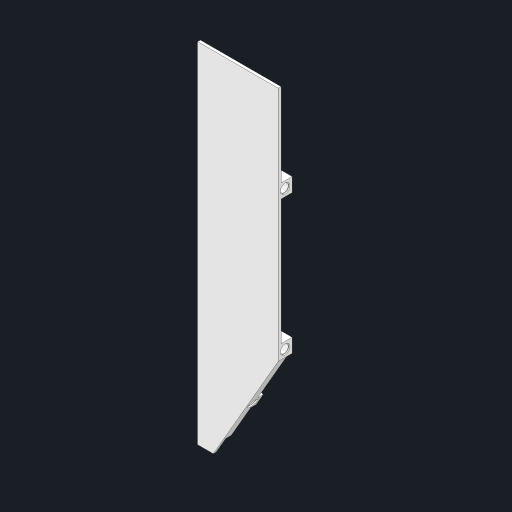
# Autodesk Inventor part: blank_side_r
Saved by Autodesk Inventor 2023 (Build 270158000, 158)
## iProperties
Created: 2024-05-25
Part Number: blank_side_r
Material: ABS Plastic
Document SubType Name: Modeling
Designer: szymo
Density: 1.06 g/cm^3
Appearance: Smooth - White
Mass: 11.6774 g
Surface Area: 101.879 cm^2
Volume: 11.0164 cm^3
Author: szymo
Autodesk Inventor part; units mm, degrees
ref_plane "YZ Plane" through (0, 0, 0) normal (1, 0, 0) x (0, 1, 0)
ref_plane "XZ Plane" through (0, 0, 0) normal (0, 1, 0) x (-1, 0, 0)
ref_plane "XY Plane" through (0, 0, 0) normal (0, 0, 1) x (1, 0, 0)
sketch "Sketch1" plane through (0, 0, 0) normal (0, 0, 1) x (1, 0, 0)
  line L0 (3.5, 3.5) -> (-1, 3.5) projected
  line L1 (-1, 3.5) -> (-1, -0.5) projected
  line L2 (-1, -0.5) -> (-4.5, -0.5) projected
  line L3 (-4.5, -0.5) -> (-4.5, -14.5) projected
  line L4 (-4.5, -14.5) -> (4.5, -0.5) projected
  line L5 (4.5, -0.5) -> (3.5, -0.5) projected
  line L6 (3.5, -0.5) -> (3.5, 3.5) projected
  circle A0 centre (13, 116) radius 15 projected
  line L7 (3.5, 3.5) -> (28, 45.9352)
  line L8 (28, 45.9352) -> (28, 131)
  line L9 (28, 131) -> (-1, 131)
  line L10 (-1, 131) -> (-1, 3.5)
  line L11 (-1, 5.5) -> (4.6547, 5.5)
  point P0 (0, 0)
  dimension "d1" = 30
  dimension "d7" = 2
  constraints: 10 end point, 2 horizontal, 2 point on line, 2 tangent, 2 vertical
  measures "d1" angle of L6 L7
  measures "d7" distance between parallel lines of L11 L0
extrude "Extrusion1" add sketch "Sketch1" against normal blind 1 contours L11 L10 A0 L8 L7 | L10 A0 | A0 L9 L8 | L10 L9 A0 picked at (14.8903, 120.4447)
sketch "Sketch3" plane through (0, 0, -1) normal (0, 0, -1) x (-1, 0, 0)
  line L0 (1, 13.25) -> (1, 15.75) projected
  line L1 (1, 15.75) -> (-2.9023, 15.75)
  line L2 (-2.9023, 15.75) -> (-2.9023, 13.25)
  line L3 (-2.9023, 13.25) -> (1, 13.25)
  line L4 (1, 13.25) -> (1, 15.75)
  line L5 (1, 5.5) -> (1, 131) projected
  line L6 (1, 11.5) -> (-4, 11.5)
  line L7 (-4, 11.5) -> (-4, 17.5)
  line L8 (-4, 17.5) -> (1, 17.5)
  line L9 (1, 17.5) -> (1, 11.5)
  line L10 (-4.6547, 5.5) -> (1, 5.5) projected
  line L11 (1, 5.5) -> (1, 131) projected
  line L12 (1, 131) -> (-28, 131) projected
  line L13 (-28, 131) -> (-28, 45.9352) projected
  line L14 (-28, 45.9352) -> (-4.6547, 5.5) projected
  line L15 (1, 20.5) -> (1, 3.5) projected
  line L16 (-4, 17.5) -> (1, 17.5)
  line L17 (1, 17.5) -> (1, 26.5)
  line L18 (1, 26.5) -> (-4, 26.5)
  line L19 (-4, 26.5) -> (-4, 17.5)
  point P0 (0, 0)
  point P1 (-2.9023, 14.5)
  point P2 (1, 17.5)
  dimension "d8" = 3
  dimension "d9" = 3
  dimension "d10" = 5
  dimension "d11" = 6
  constraints: 24 end point, 6 parallel, 3 horizontal, 3 perpendicular, 3 point on line, 1 midpoint, 1 other
  measures "d8" distance from line of L6 point (-2.902, 14.5)
  measures "d9" distance from line of L8 point (-2.902, 14.5)
  measures "d10" distance between parallel lines of L5 L7
  measures "d11" distance from line of L18 point (1, 20.5)
extrude "Extrusion2" add sketch "Sketch3" along normal blind 12 contours L3 L2 L1 L0 | L5 L6 L7 L8 L1 L2 L3
sketch "Sketch4" plane through (0, 0, -1) normal (0, 0, -1) x (-1, 0, 0)
  line L0 (-4, 11.5) -> (-4, 17.5) projected
  line L1 (1, 17.5) -> (1, 131) projected
  line L2 (1, 131) -> (-28, 131) projected
  line L3 (-28, 131) -> (-28, 45.9352) projected
  line L4 (-28, 45.9352) -> (-4.6547, 5.5) projected
  line L5 (-4.6547, 5.5) -> (1, 5.5) projected
  line L6 (1, 5.5) -> (1, 11.5) projected
  line L7 (-28, 45.9352) -> (-28, 50.9352)
  line L8 (-28, 50.9352) -> (-23, 50.9352)
  line L9 (-23, 50.9352) -> (-23, 45.9352)
  line L10 (-23, 45.9352) -> (-28, 45.9352)
  circle A0 centre (-13, 116) radius 15 projected
  line L11 (1, 131) -> (1, 5.5) projected
  line L12 (1, 101) -> (-28, 101)
  line L13 (-28, 101) -> (-23, 101)
  line L14 (-23, 101) -> (-23, 96)
  line L15 (-23, 96) -> (-28, 96)
  line L16 (-28, 96) -> (-28, 101)
  line L17 (-17.5774, 27.8827) -> (-15.0774, 23.5526)
  line L18 (-15.0774, 23.5526) -> (-10.7472, 26.0526)
  line L19 (-10.7472, 26.0526) -> (-13.2472, 30.3827)
  line L20 (-13.2472, 30.3827) -> (-17.5774, 27.8827)
  line L21 (1, 11.5) -> (-4, 11.5) projected
  line L22 (-4, 17.5) -> (1, 17.5) projected
  line L23 (1, 101) -> (-4, 101)
  line L24 (-4, 101) -> (-4, 96)
  line L25 (-4, 96) -> (1, 96)
  line L26 (1, 96) -> (1, 101)
  line L27 (1, 17.5) -> (-4, 17.5) projected
  line L28 (-4, 17.5) -> (-4, 11.5) projected
  line L29 (-4, 11.5) -> (1, 11.5) projected
  line L30 (1, 11.5) -> (1, 17.5) projected
  line L31 (1, 17.5) -> (-4, 17.5)
  line L32 (-4, 17.5) -> (-4, 22.5)
  line L33 (-4, 22.5) -> (1, 22.5)
  line L34 (1, 22.5) -> (1, 17.5)
  point P0 (0, 0)
  point P1 (1, 36.3564)
  point P2 (1, 96)
  dimension "d16" = 5
  dimension "d17" = 5
  dimension "d18" = 5
  dimension "d19" = 5
  dimension "d20" = 5
  dimension "d21" = 5
  dimension "d22" = 18.0526
  dimension "d23" = 18.0526
  dimension "d168" = 5
  dimension "d169" = 5
  dimension "d170" = 5
  dimension "d171" = 5
  constraints: 42 end point, 10 parallel, 5 perpendicular, 5 point on line, 4 horizontal, 1 tangent
  measures "d16" distance of L3.end L7.end
  measures "d17" distance of L7.end L8.end
  measures "d18" distance of L14.end L15.end
  measures "d19" distance of L13.end L14.end
  measures "d20" distance of L17.start L17.end
  measures "d21" distance of L18.end L17.end
  measures "d22" vertical distance of L17.end L4.end
  measures "d23" vertical distance of L3.end L17.start
  measures "d168" distance of L25.end L24.end
  measures "d169" distance of L24.end L23.end
  measures "d170" distance of L32.end L33.end
  measures "d171" distance of L31.end L32.end
extrude "forInserts" add sketch "Sketch4" along normal blind 4 contours L32 L33 L1 L22 | L25 L24 L12 L1 | L4 L20 L19 L18 | L3 L8 L9 L10 | L14 L15 L3 L12
sketch "Sketch5" plane through (0, 0, -1) normal (0, 0, -1) x (-1, 0, 0)
  line L0 (-28, 96) -> (-28, 50.9352) projected
  line L1 (-28, 50.9352) -> (-23, 50.9352) projected
  line L2 (-23, 50.9352) -> (-23, 45.9352) projected
  line L3 (-23, 45.9352) -> (-28, 45.9352) projected
  line L4 (-28, 45.9352) -> (-17.5774, 27.8827) projected
  line L5 (-17.5774, 27.8827) -> (-13.2472, 30.3827) projected
  line L6 (-13.2472, 30.3827) -> (-10.7472, 26.0526) projected
  line L7 (-10.7472, 26.0526) -> (-15.0774, 23.5526) projected
  line L8 (-15.0774, 23.5526) -> (-4.6547, 5.5) projected
  line L9 (-4.6547, 5.5) -> (1, 5.5) projected
  line L10 (1, 5.5) -> (1, 11.5) projected
  line L11 (-4, 11.5) -> (-4, 22.5) projected
  line L12 (1, 101) -> (1, 131) projected
  line L13 (1, 131) -> (-28, 131) projected
  line L14 (-28, 45.9352) -> (1, 45.9352)
  line L15 (1, 131) -> (1, 5.5) projected
  line L16 (-23, 50.9352) -> (1, 50.9352)
  arc A0 (-28, 101) -> (-26.5929, 101.3416) centre (-28, 104.0688) ccw
  line L17 (-28, 96) -> (1, 96)
  line L18 (-28, 101) -> (1, 101)
  line L19 (-23, 50.9352) -> (-23, 96)
  line L20 (-2, 96) -> (-2, 17.5)
  line L21 (-4, 11.5) -> (-8.1188, 11.5)
  line L22 (-2.3453, 11.5) -> (-22.2265, 45.9352)
  line L23 (-13.2472, 30.3827) -> (-2, 45.9352) construction
  line L24 (-11.8776, 28.0104) -> (-2, 41.669)
  line L25 (-5.0852, 45.9352) -> (-14.6169, 32.755)
  line L26 (1, 11.5) -> (-4, 11.5) projected
  line L27 (-28, 101) -> (-23, 101) projected
  line L28 (-23, 101) -> (-23, 96) projected
  line L29 (-23, 96) -> (-28, 96) projected
  line L30 (-4, 22.5) -> (1, 22.5) projected
  line L31 (1, 22.5) -> (1, 96) projected
  line L32 (1, 96) -> (-4, 96) projected
  line L33 (-4, 96) -> (-4, 101) projected
  line L34 (-4, 101) -> (1, 101) projected
  line L35 (-28, 131) -> (-28, 101) projected
  point P0 (0, 0)
  point P1 (1, 36.3564)
  point P2 (-2, 50.9352)
  point P3 (1, 101)
  point P4 (-4, 14.366)
  point P5 (1, 96)
  point P6 (1, 45.9352)
  point P7 (1, 101)
  point P8 (1, 45.9352)
  point P9 (-2, 22.5)
  point P10 (1, 50.9352)
  point P11 (1, 50.9352)
  dimension "d26" = 5
  dimension "d27" = 3
  dimension "d28" = 5
  dimension "d29" = 2.5
  dimension "d30" = 2.5
  constraints: 22 end point, 15 point on line, 4 parallel, 4 perpendicular, 2 point on circle, 1 centre point, 1 horizontal, 1 vertical
  measures "d26" distance between parallel lines of L14 L16
  measures "d27" distance between parallel lines of L20 L15
  measures "d28" distance between parallel lines of L4 L22
  measures "d29" distance between parallel lines of L23 L25
  measures "d30" distance between parallel lines of L23 L24
extrude "zeberka" add sketch "Sketch5" along normal blind 2 contours L28 L18 L33 L17 | L16 L20 L14 L2 | L14 L22 L5 L4 L3 | L20 L17 L15 L16 | L16 L15 L14 L20 | L20 L24 L6 L22 L25 L14 | L14 L15 L30 L20 | L15 L26 L22 L11 L30 | L22 L11 L21 L8 L7
sketch "Sketch9" plane through (-1, 5.5, 0) normal (-1, 0, 0) x (0, 0, 1)
  circle A0 centre (-9.5, 9) radius 1.25 projected
  point P0 (0, -5.5)
  constraints: 1 coincident
hole "Hole3" at (-1, 14.5, -9.5) direction (1, 0, 0) diameter 3 depth 4 counterbore diameter 3.5 counterbore depth 1
ref_plane "Work Plane1" through (-1, 91.5, -89) normal (1, 0, 0) x (0, 1, 0)
ref_plane "Work Plane2" through (-1, 91.5, -89) normal (1, 0, 0) x (0, 1, 0)
sketch "Sketch23" plane through (-1, 5.5, 0) normal (-1, 0, 0) x (0, 0, 1)
  circle A0 centre (-9.5, 9) radius 1.75 projected
  line L0 (-3, 17) -> (-5, 17) projected
  line L1 (-5, 12) -> (-5, 17) projected
  line L2 (-5, 12) -> (-13, 12) projected
  line L3 (-13, 6) -> (-13, 12) projected
  line L4 (-1, 6) -> (-13, 6) projected
  line L5 (-1, 0) -> (-1, 6) projected
  line L6 (0, 0) -> (-1, 0) projected
  line L7 (0, 125.5) -> (0, 0) projected
  line L8 (0, 125.5) -> (-1, 125.5) projected
  line L9 (-1, 95.5) -> (-1, 125.5) projected
  line L10 (-1, 95.5) -> (-5, 95.5) projected
  line L11 (-5, 90.5) -> (-5, 95.5) projected
  line L12 (-3, 90.5) -> (-5, 90.5) projected
  line L13 (-3, 17) -> (-3, 90.5) projected
  line L14 (-5, 17) -> (0, 17)
  line L15 (0, 17) -> (0, 12)
  line L16 (0, 12) -> (-5, 12)
  line L17 (-5, 12) -> (-5, 17)
  line L18 (-3, 90.5) -> (-5, 90.5) projected
  line L19 (-5, 90.5) -> (0, 90.5)
  line L20 (0, 90.5) -> (0, 95.5)
  line L21 (0, 95.5) -> (-5, 95.5)
  line L22 (-5, 95.5) -> (-5, 90.5)
  line L23 (0, 17) -> (-5, 12)
  line L24 (-5, 17) -> (-0.2081, 12.2081)
  line L25 (-5, 90.5) -> (-5, 95.5) projected
  line L26 (-5, 90.5) -> (0, 95.5)
  line L27 (-5, 95.5) -> (0, 90.5)
  point P0 (0, -5.5)
  point P1 (-2.5, 93)
  point P2 (-2.5, 14.5)
  dimension "d172" = 5
  dimension "d173" = 5
  dimension "d174" = 5
  dimension "d175" = 5
  constraints: 24 end point, 4 parallel, 3 perpendicular, 2 horizontal, 2 midpoint, 1 point on line
  measures "d172" distance of L15.end L16.end
  measures "d173" distance of L14.end L15.end
  measures "d174" distance of L21.end L20.end
  measures "d175" distance of L20.end L19.end
hole "Hole8" at (-1, 98.5, -2.5) at (-1, 20, -2.5) direction (1, 0, 0) diameter 3 depth 4.9 counterbore diameter 3.5 counterbore depth 0.4
sketch "Sketch24" plane through (28, 45.9352, 0) normal (1, 0, 0) x (0, 0, -1)
  line L0 (0, 0) -> (0, 85.0648) projected
  line L1 (0, 0) -> (3, 0) projected
  line L2 (3, 0) -> (5, 0) projected
  line L3 (5, 5) -> (5, 0) projected
  line L4 (1, 5) -> (5, 5) projected
  line L5 (1, 50.0648) -> (1, 5) projected
  line L6 (1, 50.0648) -> (5, 50.0648) projected
  line L7 (5, 55.0648) -> (5, 50.0648) projected
  line L8 (1, 55.0648) -> (5, 55.0648) projected
  line L9 (1, 85.0648) -> (1, 55.0648) projected
  line L10 (0, 85.0648) -> (1, 85.0648) projected
  line L11 (5, 5) -> (0, 5)
  line L12 (0, 5) -> (0, 0)
  line L13 (0, 0) -> (5, 0)
  line L14 (5, 0) -> (5, 5)
  line L15 (5, 50.0648) -> (5, 55.0648) projected
  line L16 (5, 50.0648) -> (0, 50.0648)
  line L17 (0, 50.0648) -> (0, 55.0648)
  line L18 (0, 55.0648) -> (5, 55.0648)
  line L19 (5, 55.0648) -> (5, 50.0648)
  line L20 (5, 5) -> (0, 0)
  line L21 (0, 5) -> (5, 0)
  line L22 (5, 55.0648) -> (0, 50.0648)
  line L23 (0, 55.0648) -> (5, 50.0648)
  point P0 (0, -45.9352)
  point P1 (2.5, 2.5)
  point P2 (2.5, 52.5648)
  dimension "d183" = 5
  dimension "d184" = 5
  constraints: 24 end point, 4 parallel, 4 perpendicular, 2 horizontal, 2 midpoint, 1 point on line
  measures "d183" distance of L17.end L18.end
  measures "d184" distance of L16.end L17.end
hole "Hole9" at (28, 48.4352, -2.5) at (28, 98.5, -2.5) direction (-1, 0, 0) diameter 3 depth 4.9 counterbore diameter 3.5 counterbore depth 0.4
sketch "Sketch25" plane through (28, 45.9352, 0) normal (0.8660254, -0.5, 0) x (0, 0, -1)
  line L0 (0, -46.6906) -> (0, 0) projected
  line L1 (0, -46.6906) -> (1, -46.6906) projected
  line L2 (1, -39.7624) -> (1, -46.6906) projected
  line L3 (1, -39.7624) -> (3, -39.7624) projected
  line L4 (3, -25.8453) -> (3, -39.7624) projected
  line L5 (3, -25.8453) -> (5, -25.8453) projected
  line L6 (5, -20.8453) -> (5, -25.8453) projected
  line L7 (3, -20.8453) -> (5, -20.8453) projected
  line L8 (3, 0) -> (3, -20.8453) projected
  line L9 (0, 0) -> (3, 0) projected
  line L10 (5, -20.8453) -> (0, -20.8453)
  line L11 (0, -20.8453) -> (0, -25.8453)
  line L12 (0, -25.8453) -> (5, -25.8453)
  line L13 (5, -25.8453) -> (5, -20.8453)
  line L14 (5, -25.8453) -> (0, -20.8453)
  line L15 (5, -20.8453) -> (0, -25.8453)
  point P0 (0, -53.7811)
  point P1 (2.5, -23.3453)
  dimension "d193" = 5
  dimension "d194" = 5
  constraints: 12 end point, 2 parallel, 2 perpendicular, 1 horizontal, 1 midpoint
  measures "d193" distance of L12.end L11.end
  measures "d194" distance of L11.end L10.end
hole "Hole10" at (16.3274, 25.7176, -2.5) direction (-0.8660254, 0.5, 0) diameter 3 depth 4.9 counterbore diameter 3.5 counterbore depth 0.4
equation "\"d22\" = d23"
body "Solid1"
